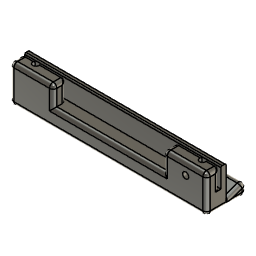
plate attacment v3 v1 (Autodesk Fusion 360 design; units mm, degrees)
Autodesk Fusion 360 part; units mm, degrees
sketch "Sketch1" plane through (0, 0, 0) normal (0, 0, 1) x (1, 0, 0)
  line L0 (0, 0) -> (15, 0)
  line L1 (15, 0) -> (15, 16)
  line L2 (15, 16) -> (0, 16)
  line L3 (0, 16) -> (0, 0)
  line L4 (0, 16) -> (15, 16) construction
  line L5 (15, 16) -> (15, 8) construction
  line L6 (15, 8) -> (0, 8) construction
  line L7 (0, 8) -> (0, 16) construction
  line L8 (0, 8) -> (0, 5.9) construction
  line L9 (0, 5.9) -> (8, 5.9)
  line L10 (8, 5.9) -> (8, 5.15)
  line L11 (8, 5.15) -> (0, 5.15)
  line L12 (0, 5.15) -> (0, 5.9)
  line L13 (9.9062, 16) -> (9.9062, 8)
  line L14 (0, 8) -> (9.9062, 8)
  line L15 (15.0938, 10.0608) -> (9.9062, 8)
  line L16 (9.9062, 16) -> (12.5, 9.0304)
  dimension "d1" = 15
  dimension "d2" = 16
  dimension "d3" = 15
  dimension "d4" = 8
  dimension "d5" = 2.1
  dimension "d6" = 8
  dimension "d7" = 0.75
  dimension "d32" = 2.5
  constraint horizontal L0
  constraint vertical L1
  constraint horizontal L2
  constraint vertical L3
  constraint coincident L0.start L3.end
  constraint horizontal L4
  constraint vertical L5
  constraint horizontal L6
  constraint vertical L7
  constraint perpendicular L6 L8
  constraint horizontal L9
  constraint vertical L10
  constraint horizontal L11
  constraint vertical L12
  constraint coincident L2 L13.start
  constraint coincident L6 L13.end
  constraint perpendicular L6 L13
  constraint midpoint L15 L16.end
  measures "d1" distance of L0.start L0.end
  measures "d2" distance of L0.start L2.end
  measures "d3" distance of L2.end L1.end
  measures "d4" distance of L2.end L6.end
  measures "d5" distance of L6.end L8.end
  measures "d6" distance of L8.end L9.end
  measures "d7" distance of L8.end L11.end
  measures "d32" distance of L1 L16.end
extrude "Extrude1" add sketch "Sketch1" along normal blind 80 contours L0 L1 L3 L9 L10 L11 L14 L15 | L1 L2 L15 L16
sketch "Sketch2" plane through (15, 0, 0) normal (1, 0, 0) x (0, 1, 0)
  line L0 (0, 0) -> (16, 0)
  line L1 (16, 0) -> (16, 80)
  line L2 (16, 80) -> (0, 80)
  line L3 (0, 80) -> (0, 0)
  line L4 (0, 40) -> (16, 40) construction
  line L5 (9.03, 47.5) -> (16, 47.5)
  line L6 (16, 47.5) -> (16, 32.5)
  line L7 (16, 32.5) -> (9.03, 32.5)
  line L8 (9.03, 32.5) -> (9.03, 47.5)
  line L9 (9.03, 40) -> (16, 40) construction
  dimension "d10" = 6.97
  dimension "d11" = 15
  constraint midpoint L3 L4.start
  constraint midpoint L1 L4.end
  constraint horizontal L5
  constraint vertical L6
  constraint horizontal L7
  constraint vertical L8
  constraint midpoint L8 L9.start
  constraint midpoint L6 L4.end
  constraint collinear L4 L9
  constraint collinear L1 L6
  measures "d10" distance of L5.start L5.end
  measures "d11" distance of L5.start L7.end
extrude "Extrude2" cut sketch "Sketch2" against normal blind 7 contours L1 L5 L6 L7 L8
chamfer "Chamfer1" distance 6.97 angle 45 2 edges at (12.4531, 16, 47.5) (12.4531, 16, 32.5)
fillet "Fillet2" radius 0.5 3 edges at (0, 5.15, 40) (0, 5.9, 40) (0, 8, 40)
sketch "Sketch4" plane through (15, 0, 0) normal (1, 0, 0) x (0, 1, 0)
  line L0 (16, 25.53) -> (9.03, 32.5)
  line L1 (9.03, 32.5) -> (9.03, 47.5)
  line L2 (9.03, 47.5) -> (16, 54.47)
  line L3 (16, 54.47) -> (16, 80)
  line L4 (16, 80) -> (0, 80)
  line L5 (0, 80) -> (0, 0)
  line L6 (0, 0) -> (16, 0)
  line L7 (16, 0) -> (16, 25.53)
  circle A0 centre (4.4, 74) radius 1.25
  circle A1 centre (4.4, 74) radius 2.75
  line L8 (0, 40) -> (9.03, 40) construction
  circle A2 centre (4.4, 6) radius 1.25
  circle A3 centre (4.4, 6) radius 2.75
  dimension "d33" = 2.5
  dimension "d34" = 4.4
  dimension "d37" = 5.5
  dimension "d40" = 6
  constraint concentric A0 A1
  constraint midpoint L5 L8.start
  constraint midpoint L1 L8.end
  constraint symmetric A0 L8 A2
  constraint symmetric A1 L8 A3
  measures "d33" diameter of A0
  measures "d34" distance of L5 A0.centre
  measures "d37" diameter of A1
  measures "d40" distance of L4 A0.centre
extrude "Extrude7" cut sketch "Sketch4" against normal blind 17 contours A0 | A2
extrude "Extrude8" cut sketch "Sketch4" against normal blind 5.5 contours A1 | A3
sketch "Sketch5" plane through (0, 0, 0) normal (0, -1, 0) x (1, 0, 0)
  line L0 (0, 0) -> (15, 0)
  line L1 (15, 0) -> (15, 80)
  line L2 (15, 80) -> (0, 80)
  circle A0 centre (4.5, 71.5) radius 1.25
  line L3 (0, 80) -> (0, 0)
  line L4 (15, 40) -> (0, 40) construction
  line L5 (0, 62.5) -> (8, 62.5)
  line L6 (8, 62.5) -> (8, 17.5)
  line L7 (8, 17.5) -> (0, 17.5)
  line L8 (0, 17.5) -> (0, 62.5)
  line L9 (0, 40) -> (8, 40) construction
  dimension "d45" = 2.5
  dimension "d46" = 8.5
  dimension "d47" = 4.5
  dimension "d51" = 8
  dimension "d52" = 45
  constraint midpoint L1 L4.start
  constraint midpoint L3 L4.end
  constraint horizontal L5
  constraint vertical L6
  constraint horizontal L7
  constraint vertical L8
  constraint coincident L3 L5.start
  constraint midpoint L8 L4.end
  constraint midpoint L6 L9.end
  constraint collinear L4 L9
  measures "d45" diameter of A0
  measures "d46" distance of L2 A0.centre
  measures "d47" distance of A0.centre L3
  measures "d51" distance of L5.start L5.end
  measures "d52" distance of L5.start L7.end
extrude "Extrude9" cut sketch "Sketch5" against normal blind 11 contours A0
chamfer "Chamfer2" distance 1.5 angle 45 2 edges at (9.5, 3.2346, 5.548) (9.5, 3.2346, 73.548)
extrude "Extrude10" cut sketch "Sketch5" against normal blind 5.15 contours L3 L5 L6 L7 L8
fillet "Fillet4" radius 1.5 32 edges at (4.25, 5.15, 80) (0.1464, 5.0036, 80) (0, 2.325, 80) (7.5, 0, 80) (4.25, 5.15, 62.5) (0.1464, 5.0036, 62.5) (0, 2.325, 62.5) (0, 0, 71.25) (4, 0, 62.5) (8, 0, 40) (15, 0, 40) (0, 2.325, 17.5) (0.1464, 5.0036, 17.5) (4.25, 5.15, 17.5) (4, 0, 17.5) (0, 0, 8.75) (7.5, 0, 0) (4.25, 5.15, 0) (0.1464, 5.0036, 0) (0, 2.325, 0) (15, 8, 80) (15, 8, 0) (15, 16, 67.235) (15, 16, 12.765) (9.9062, 16, 67.235) (9.9062, 16, 12.765) (11.2031, 12.5152, 80) (11.2031, 8.5152, 80) (12.4531, 16, 80) (11.2031, 8.5152, 0) (11.2031, 12.5152, 0) (12.4531, 16, 0)
move_body "Move1" bodies 1 to x (0, 0, -1) y (0, 1, 0) z (1, 0, 0) at (0, 0, -0.0057)
